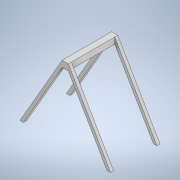
# Autodesk Inventor part: stativ ide 1
Saved by Autodesk Inventor 2022 (Build 260153000, 153)
## iProperties
Created: 2022-04-04
Part Number: stativ ide 1
Material: Generic
Document SubType Name: Modeling
Designer: tigri
Density: 1 g/cm^3
Appearance: Default
Author: tigri
Autodesk Inventor part; units mm, degrees
ref_plane "YZ Plane" through (0, 0, 0) normal (1, 0, 0) x (0, 1, 0)
ref_plane "XZ Plane" through (0, 0, 0) normal (0, 1, 0) x (-1, 0, 0)
ref_plane "XY Plane" through (0, 0, 0) normal (0, 0, 1) x (1, 0, 0)
sketch "Sketch1" plane through (0, 0, 0) normal (0, 0, 1) x (1, 0, 0)
  point P0 (0, 0)
sketch "Sketch2" plane through (0, 0, 0) normal (0, 0, 1) x (1, 0, 0)
  line L0 (0, 650) -> (375.2777, 0)
  line L1 (409.9187, 0) -> (375.2777, 0)
  line L2 (409.9187, 0) -> (0, 710)
  line L3 (0, 650) -> (0, 710)
  point P0 (0, 0)
  dimension "d0" = 650
  constraints: 8 end point, 1 horizontal, 1 parallel, 1 vertical
  measures "d0" distance of point (0, 0) L0.start
extrude "Extrusion1" add sketch "Sketch2" against normal blind 30
sketch "Sketch3" plane through (0, 0, 0) normal (0, 0, 1) x (1, 0, 0)
  line L0 (0, 650) -> (0, 710) projected
  line L1 (0, 650) -> (-60, 650)
  line L2 (-60, 650) -> (-60, 710)
  line L3 (-60, 710) -> (0, 710)
  line L4 (0, 710) -> (0, 650)
  line L5 (-60, 650) -> (-435.277, 0)
  line L6 (-60, 710) -> (-469.918, 0)
  line L7 (-469.918, 0) -> (-435.277, 0)
  point P0 (0, 0)
  dimension "d5" = 60
  dimension "d6" = 750.555
  constraints: 14 end point, 2 horizontal, 2 parallel, 1 perpendicular
  measures "d5" distance of L2.end L3.end
  measures "d6" distance of L1.end L5.end
extrude "Extrusion2" add sketch "Sketch3" against normal blind 30 contours L5 L7 L6 L2
sketch "Sketch4" plane through (0, 0, 0) normal (0, 0, 1) x (1, 0, 0)
  line L0 (0, 710) -> (409.9187, 0) projected
  line L1 (-60, 650) -> (0, 650)
  line L2 (0, 650) -> (0, 710)
  line L3 (0, 710) -> (-60, 710)
  line L4 (-60, 710) -> (-60, 650)
  point P0 (0, 0)
  constraints: 8 end point, 2 parallel, 1 horizontal, 1 perpendicular
extrude "Extrusion3" add sketch "Sketch4" against normal blind 60
sketch "Sketch5" plane through (0, 0, 0) normal (0, 0, 1) x (1, 0, 0)
  point P0 (0, 0)
sketch "Sketch6" plane through (0, 0, -60) normal (0, 0, -1) x (-1, 0, 0)
  line L0 (0, 710) -> (-409.9187, 0) projected
  line L1 (60, 650) -> (435.277, 0) projected
  line L2 (0, 710) -> (60, 710)
  line L3 (60, 710) -> (60, 650)
  line L4 (60, 650) -> (0, 650)
  line L5 (0, 650) -> (0, 710)
  point P0 (0, 0)
  constraints: 8 end point, 2 parallel, 1 horizontal, 1 perpendicular
extrude "Extrusion4" add sketch "Sketch6" along normal blind 420
sketch "Sketch7" plane through (0, 0, -480) normal (0, 0, -1) x (-1, 0, 0)
  line L0 (60, 650) -> (435.277, 0) projected
  line L1 (60, 650) -> (435.277, 0)
  line L2 (469.918, 0) -> (60, 710) projected
  line L3 (435.277, 0) -> (469.918, 0)
  line L4 (469.918, 0) -> (60, 710)
  line L5 (60, 710) -> (60, 650)
  point P0 (0, 0)
  constraints: 8 end point, 2 collinear, 1 horizontal, 1 perpendicular
extrude "Extrusion5" add sketch "Sketch7" against normal blind 30
sketch "Sketch8" plane through (0, 0, -480) normal (0, 0, -1) x (-1, 0, 0)
  line L0 (-375.2777, 0) -> (0, 650) projected
  line L1 (0, 650) -> (-375.2777, 0)
  line L2 (0, 710) -> (-409.9187, 0) projected
  line L3 (-375.2777, 0) -> (-409.9187, 0)
  line L4 (-409.9187, 0) -> (0, 710)
  line L5 (0, 710) -> (0, 650)
  point P0 (0, 0)
  constraints: 8 end point, 2 collinear, 1 horizontal, 1 perpendicular
extrude "Extrusion6" add sketch "Sketch8" against normal blind 30
body "Solid1"
